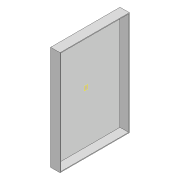
# Autodesk Inventor part: Задняя стенка
Saved by Autodesk Inventor 2022 (Build 260153000, 153)
## iProperties
Created: 2023-02-20
Part Number: Задняя стенка
Material: Типовые
Document SubType Name: Modeling
Designer: Глеб
Density: 1 g/cm^3
Appearance: По умолчанию
Author: Глеб
Autodesk Inventor part; units mm, degrees
ref_plane "YZ Plane" through (0, 0, 0) normal (1, 0, 0) x (0, 1, 0)
ref_plane "XZ Plane" through (0, 0, 0) normal (0, 1, 0) x (-1, 0, 0)
ref_plane "XY Plane" through (0, 0, 0) normal (0, 0, 1) x (1, 0, 0)
ref_plane "РабПлоскость1" through (8, 0, 0) normal (1, 0, 0) x (0, 0, -1)
sketch "Эскиз2" plane through (8, 0, 0) normal (1, 0, 0) x (0, 0, -1)
  line L0 (200, 300) -> (-200, 300) projected
  line L1 (200, -300) -> (200, 300) projected
  line L2 (-200, 300) -> (200, 300)
  line L3 (200, 300) -> (200, -300)
  line L4 (200, -300) -> (-200, -300)
  line L5 (-200, -300) -> (-200, 300)
  line L6 (-196, 296) -> (196, 296)
  line L7 (196, 296) -> (196, -296)
  line L8 (196, -296) -> (-196, -296)
  line L9 (-196, -296) -> (-196, 296)
  point P0 (0, 0)
  dimension "d4" = 4
  dimension "d5" = 4
  dimension "d6" = 4
  dimension "d7" = 4
  constraints: 16 end point, 4 parallel, 2 horizontal, 2 perpendicular
  measures "d4" distance between parallel lines of L0 L6
  measures "d5" distance between parallel lines of L1 L7
  measures "d6" distance between parallel lines of L5 L9
  measures "d7" distance between parallel lines of L8 L4
extrude "Выдавливание2" add sketch "Эскиз2" along normal blind 50
sketch "Эскиз3" plane through (8, 0, 0) normal (-1, 0, 0) x (0, 0, 1)
  line L0 (-200, -300) -> (-200, 300) projected
  line L1 (200, 300) -> (200, -300) projected
  line L2 (-200, 300) -> (200, 300)
  line L3 (200, 300) -> (200, -300)
  line L4 (200, -300) -> (-200, -300)
  line L5 (-200, -300) -> (-200, 300)
  point P0 (0, 0)
  constraints: 8 end point, 2 parallel, 1 horizontal, 1 perpendicular
extrude "Выдавливание3" add sketch "Эскиз3" along normal blind 4
equation "\"d5\" = d4"
equation "\"d6\" = d4"
equation "\"d7\" = d4"
